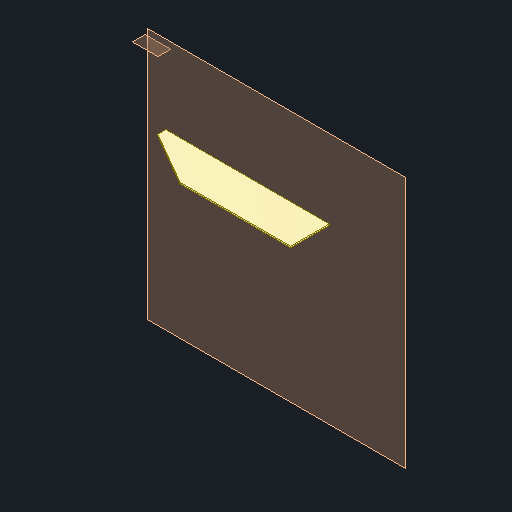
# Autodesk Inventor part: right_hold
Saved by Autodesk Inventor 2023 (Build 270158000, 158)
## iProperties
Created: 2024-05-18
Part Number: right_hold
Material: Nylon 6/6
Document SubType Name: Modeling
Designer: szymo
Density: 1.13 g/cm^3
Appearance: Nylon 6
Mass: 3.75247 g
Surface Area: 69.3814 cm^2
Volume: 3.32077 cm^3
Author: szymo
Autodesk Inventor part; units mm, degrees
ref_plane "YZ Plane" through (0, 0, 0) normal (1, 0, 0) x (0, 1, 0)
ref_plane "XZ Plane" through (0, 0, 0) normal (0, 1, 0) x (-1, 0, 0)
ref_plane "XY Plane" through (0, 0, 0) normal (0, 0, 1) x (1, 0, 0)
ref_plane "Work Plane1" through (0, 0, 0) normal (0, 0, 1) x (1, 0, 0)
sketch "Sketch1" plane through (0, 0, 0) normal (0, 0, 1) x (1, 0, 0)
  line L0 (-71, -74) -> (-71, -89) projected
  line L1 (-71, -89) -> (41, -89) projected
  line L2 (41, -89) -> (41, -30.5) projected
  line L3 (41, -30.5) -> (91, -30.5) projected
  line L4 (91, -30.5) -> (91, 30.5) projected
  line L5 (91, 30.5) -> (41, 30.5) projected
  line L6 (41, 30.5) -> (41, 89) projected
  line L7 (41, 89) -> (-71, 89) projected
  line L8 (-71, 89) -> (-71, 74) projected
  line L9 (-71, 74) -> (-87, 74) projected
  line L10 (-87, 74) -> (-87, 89) projected
  line L11 (-87, 89) -> (-91, 89) projected
  line L12 (-91, 89) -> (-91, -89) projected
  line L13 (-91, -89) -> (-87, -89) projected
  line L14 (-87, -89) -> (-87, -74) projected
  line L15 (-87, -74) -> (-71, -74) projected
  line L16 (12, 37) -> (40, 37) projected
  line L17 (41, 37) -> (-86, 37)
  line L18 (-86, 37) -> (-86, 36)
  line L19 (-86, 36) -> (41, 36)
  line L20 (41, 36) -> (41, 37)
  circle A0 centre (-83, 21.5) radius 1.2295 projected
  circle A1 centre (-83, -64.5) radius 1.2295 projected
  circle A2 centre (-83, -21.5) radius 1.2295 projected
  circle A3 centre (-83, 64.5) radius 1.2295 projected
  line L21 (-85, -72) -> (-76, -72) projected
  line L22 (-76, -72) -> (-76, -57) projected
  line L23 (-76, -57) -> (-85, -57) projected
  arc A4 (-87, -55) -> (-85, -57) centre (-85, -55) ccw projected
  line L24 (-87, -55) -> (-87, -31) projected
  arc A5 (-85, -29) -> (-87, -31) centre (-85, -31) ccw projected
  line L25 (-85, -29) -> (-76, -29) projected
  line L26 (-76, -29) -> (-76, -14) projected
  line L27 (-76, -14) -> (-85, -14) projected
  arc A6 (-87, -12) -> (-85, -14) centre (-85, -12) ccw projected
  line L28 (-87, -12) -> (-87, 12) projected
  arc A7 (-85, 14) -> (-87, 12) centre (-85, 12) ccw projected
  line L29 (-85, 14) -> (-76, 14) projected
  line L30 (-76, 14) -> (-76, 29) projected
  line L31 (-76, 29) -> (-85, 29) projected
  arc A8 (-87, 31) -> (-85, 29) centre (-85, 31) ccw projected
  line L32 (-87, 31) -> (-87, 55) projected
  arc A9 (-85, 57) -> (-87, 55) centre (-85, 55) ccw projected
  line L33 (-85, 57) -> (-76, 57) projected
  line L34 (-76, 57) -> (-76, 72) projected
  line L35 (-76, 72) -> (-85, 72) projected
  arc A10 (-87, 74) -> (-85, 72) centre (-85, 74) ccw projected
  line L36 (-87, 74) -> (-87, 89) projected
  line L37 (-91, 89) -> (-87, 89) projected
  line L38 (-91, -89) -> (-91, 89) projected
  line L39 (-91, -89) -> (-87, -89) projected
  line L40 (-87, -89) -> (-87, -74) projected
  arc A11 (-85, -72) -> (-87, -74) centre (-85, -74) ccw projected
  point P0 (0, 0)
  dimension "d1" = 0
  dimension "d2" = 1
  dimension "d11" = 1
  constraints: 8 end point, 2 parallel, 1 horizontal, 1 perpendicular, 1 point on line
  measures "d1" distance between parallel lines of L16 L17
  measures "d2" distance between parallel lines of L16 L19
  measures "d11" distance between parallel lines of L18 L32
ref_plane "Work Plane2" through (11, 8.5, 30) normal (0, 0, 1) x (1, 0, 0)
extrude "Extrusion1" add sketch "Sketch1" along normal up to surface (30 mm away) contours L19 L18 L17 L16 L6
ref_plane "Work Plane3" through (-90.5, 89, 1) normal (0, 1, 0) x (0, 0, 1)
sketch "Sketch3" plane through (-90.5, 89, 1) normal (0, 1, 0) x (0, 0, 1)
  line L0 (3.5, 3.5) -> (-1, 3.5) projected
  line L1 (-1, 3.5) -> (-1, -0.5) projected
  line L2 (-1, -0.5) -> (-4.5, -0.5) projected
  line L3 (-4.5, -0.5) -> (-4.5, -14.5) projected
  line L4 (-4.5, -14.5) -> (4.5, -0.5) projected
  line L5 (4.5, -0.5) -> (3.5, -0.5) projected
  line L6 (3.5, -0.5) -> (3.5, 3.5) projected
  line L7 (29, 4.5) -> (29, 131.5) projected
  line L8 (-1, 131.5) -> (29, 131.5) projected
  line L9 (-1, 131.5) -> (-1, 4.5) projected
  line L10 (-1, 4.5) -> (29, 4.5) projected
  line L11 (3.5, -0.5) -> (30.1547, 45.6673)
  line L12 (30.1547, 45.6673) -> (29, 45.6673)
  line L13 (29, 45.6673) -> (3.5, 1.5)
  point P0 (-1, 90.5)
  point P1 (5.2321, 4.5)
  dimension "d13" = 1
  constraints: 6 end point, 1 midpoint, 1 parallel, 1 perpendicular, 1 point on line
  measures "d13" distance between parallel lines of L13 L11
extrude "Extrusion3" cut sketch "Sketch3" against normal up to next contours L13 L7 L11 L10 | L11 L7 L10
body "Solid1"
